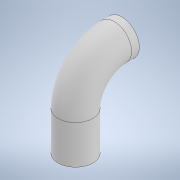
# Autodesk Inventor part: Rørende - water block
Saved by Autodesk Inventor 2020 (Build 240168000, 168)
## iProperties
Created: 2021-05-19
Part Number: Rørende - water block
Material: Generic
Document SubType Name: Modeling
Designer: 6128059
Density: 1 g/cm^3
Appearance: Default
Author: 6128059
Autodesk Inventor part; units mm, degrees
ref_plane "YZ Plane" through (0, 0, 0) normal (1, 0, 0) x (0, 1, 0)
ref_plane "XZ Plane" through (0, 0, 0) normal (0, 1, 0) x (-1, 0, 0)
ref_plane "XY Plane" through (0, 0, 0) normal (0, 0, 1) x (1, 0, 0)
sketch "Sketch1" plane through (0, 0, 0) normal (0, 1, 0) x (-1, 0, 0)
  circle A0 centre (0, 0) radius 4.5
  circle A1 centre (0, 0) radius 4.25
  dimension "d0" = 9
  dimension "d1" = 8.5
  constraints: 2 centre point, 2 coincident
  measures "d0" diameter of A0
  measures "d1" diameter of A1
sketch "Sketch2" plane through (0, 0, 0) normal (1, 0, 0) x (0, 1, 0)
  line L0 (0, 0) -> (0, -10) construction
  arc A0 (10, -10) -> (0, 0) centre (0, -10) ccw
  dimension "d2" = 10
  constraints: 2 end point, 2 point on circle, 1 centre point, 1 coincident, 1 vertical
  measures "d2" distance of L0.start L0.end
extrude "Extrusion1" add sketch "Sketch1" against normal blind 10
sketch "Sketch3" plane through (0, 0, 0) normal (0, 1, 0) x (1, 0, 0)
  circle A0 centre (0, 0) radius 4.25 projected
  circle A1 centre (0, 0) radius 4.5 projected
sweep "Sweep1" add profiles "Sketch3" path "Sketch2"
sketch "Sketch4" plane through (0, 10, -10) normal (0, 0, -1) x (-1, 0, 0)
  circle A0 centre (0, 0) radius 4.25 projected
  circle A1 centre (0, 0) radius 4.5 projected
  point P0 (0, -10)
extrude "Extrusion2" add sketch "Sketch4" along normal blind 2
body "Solid1"
